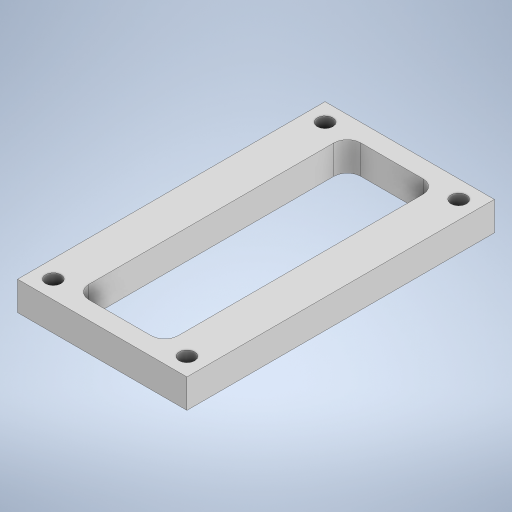
# Autodesk Inventor part: RectangularHolderFloor
Saved by Autodesk Inventor 2024 (Build 280153000, 153)
## iProperties
Created: 2023-08-14
Part Number: RectangularHolderFloor
Material: Generic
Document SubType Name: Modeling
Designer: ewinden
Density: 1 g/cm^3
Appearance: Default
Author: ewinden
Autodesk Inventor part; units mm, degrees
ref_plane "YZ Plane" through (0, 0, 0) normal (1, 0, 0) x (0, 1, 0)
ref_plane "XZ Plane" through (0, 0, 0) normal (0, 1, 0) x (-1, 0, 0)
ref_plane "XY Plane" through (0, 0, 0) normal (0, 0, 1) x (1, 0, 0)
sketch "Sketch1" plane through (0, 0, 0) normal (0, 1, 0) x (-1, 0, 0)
  line L0 (0, 0) -> (38, 0)
  line L1 (38, 0) -> (38, -69)
  line L2 (38, -69) -> (0, -69)
  line L3 (0, -69) -> (0, 0)
  line L4 (12, -4) -> (26, -4)
  line L5 (29, -7) -> (29, -62)
  line L6 (26, -65) -> (12, -65)
  line L7 (9, -62) -> (9, -7)
  arc A0 (29, -7) -> (26, -4) centre (26, -7) ccw
  arc A1 (12, -4) -> (9, -7) centre (12, -7) ccw
  arc A2 (9, -62) -> (12, -65) centre (12, -62) ccw
  arc A3 (26, -65) -> (29, -62) centre (26, -62) ccw
  dimension "d0" = 38
  dimension "d1" = 69
  dimension "d2" = 4
  dimension "d3" = 9
  dimension "d4" = 4
  dimension "d5" = 9
  dimension "d6" = 3
  constraints: 16 end point, 8 point on circle, 8 tangent, 4 centre point, 4 parallel, 3 equal radius, 2 horizontal, 2 perpendicular
  measures "d0" distance of L0.start L0.end
  measures "d1" distance of L2.end L0.start
  measures "d2" distance between parallel lines of L0 L4
  measures "d3" distance between parallel lines of L1 L5
  measures "d4" distance between parallel lines of L2 L6
  measures "d5" distance between parallel lines of L7 L3
  measures "d6" radius of A0
extrude "Extrusion1" add sketch "Sketch1" along normal blind 6.5
sketch "Sketch2" plane through (0, 0, 0) normal (0, -1, 0) x (1, 0, 0)
  line L0 (-34, -65) -> (-4, -65) construction
  line L1 (-4, -65) -> (-4, -4) construction
  line L2 (-4, -4) -> (-34, -4) construction
  line L3 (-34, -4) -> (-34, -65) construction
  circle A0 centre (-34, -4) radius 1.75
  circle A1 centre (-4, -4) radius 1.75
  circle A2 centre (-4, -65) radius 1.75
  circle A3 centre (-34, -65) radius 1.75
  line L4 (-38, -69) -> (-38, 0) projected
  line L5 (-38, 0) -> (0, 0) projected
  line L6 (0, 0) -> (0, -69) projected
  line L7 (0, -69) -> (-38, -69) projected
  dimension "d9" = 3.5
  dimension "d10" = 4
  dimension "d11" = 4
  dimension "d12" = 4
  dimension "d13" = 4
  constraints: 8 end point, 4 centre point, 4 coincident, 3 equal radius, 2 parallel, 1 horizontal, 1 perpendicular
  measures "d9" diameter of A0
  measures "d10" distance between parallel lines of L4 L3
  measures "d11" distance between parallel lines of L5 L2
  measures "d12" distance between parallel lines of L6 L1
  measures "d13" distance between parallel lines of L7 L0
extrude "Extrusion2" cut sketch "Sketch2" against normal blind 6.5 contours A0 | A1 | A2 | A3
equation "\"d4\" = d2"
equation "\"d5\" = d3"
equation "\"d11\" = d10"
equation "\"d12\" = d10"
equation "\"d13\" = d10"
body "Solid1"
